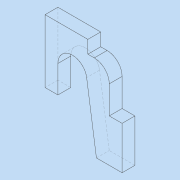
# Autodesk Inventor part: 0 零件
Saved by Autodesk Inventor 2020 (Build 240168000, 168)
## iProperties
Created: 2020-11-03
Part Number: 0 零件
Material: 一般
Document SubType Name: Modeling
Designer: p2013
Density: 1 g/cm^3
Appearance: 預設
Author: p2013
Autodesk Inventor part; units mm, degrees
ref_plane "YZ Plane" through (0, 0, 0) normal (1, 0, 0) x (0, 1, 0)
ref_plane "XZ Plane" through (0, 0, 0) normal (0, 1, 0) x (-1, 0, 0)
ref_plane "XY Plane" through (0, 0, 0) normal (0, 0, 1) x (1, 0, 0)
sketch "草圖1" plane through (0, 0, 0) normal (0, 0, 1) x (1, 0, 0)
  line L0 (0, 0) -> (8.1318, 0) construction
  line L1 (0, 0) -> (0, 16.2395) construction
  line L2 (-3.5, 0) -> (-15, 0)
  line L3 (-15, 0) -> (-15, -12)
  line L4 (-15, -12) -> (-13, -12)
  line L5 (-13, -12) -> (-13, -4)
  line L6 (0, -10) -> (0, -3.5)
  line L7 (0, -10) -> (3, -10)
  line L8 (3, -10) -> (3, -5)
  line L9 (3, -5) -> (0, -5)
  line L10 (0, -5) -> (0, -10)
  line L11 (-15, 0) -> (-5, 0)
  line L12 (-5, 0) -> (-5, 3)
  line L13 (-5, 3) -> (-15, 3)
  line L14 (-15, 3) -> (-15, 0)
  arc A0 (-9.5042, -2.6723) -> (-13, -4) centre (-11, -4) ccw
  line L15 (-9.5042, -2.6723) -> (-3, -10)
  line L16 (-3, -10) -> (0, -10)
  arc A1 (0, -3.5) -> (-3.5, 0) centre (-3.5, -3.5) ccw
  point P0 (0, -5)
  point P1 (-5, 0)
  dimension "d0" = 2
  dimension "d1" = 3
  dimension "d2" = 3
  dimension "d3" = 15
  dimension "d6" = 5
  dimension "d7" = 3.5
  dimension "d8" = 10
  dimension "d9" = 10
  dimension "d15" = 12
  dimension "d16" = 8
  dimension "d17" = 2
  dimension "d18" = 3
  constraints: 34 end point, 4 horizontal, 4 parallel, 4 perpendicular, 4 point on circle, 4 tangent, 3 point on line, 3 vertical, 2 centre point
  measures "d0" distance between parallel lines of L3 L5
  measures "d1" distance between parallel lines of L2 L13
  measures "d2" distance between parallel lines of L10 L8
  measures "d3" distance between parallel lines of L6 L3
  measures "d6" distance between parallel lines of L7 L9
  measures "d7" radius of A1
  measures "d8" distance between parallel lines of L14 L12
  measures "d9" distance between parallel lines of L2 L7
  measures "d15" distance between parallel lines of L2 L4
  measures "d16" distance of L4.end L5.end
  measures "d17" radius of A0
  measures "d18" distance of L15.end L6.start
extrude "擠出1" add sketch "草圖1" along normal mid plane 3
equation "\"d2\" = d1"
